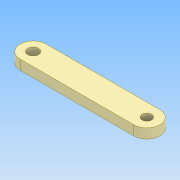
# Autodesk Inventor part: Selection_Counterweight
Saved by Autodesk Inventor 2018.1 (Build 221171000, 171)
## iProperties
Created: 2019-02-14
Part Number: Selection_Counterweight
Material: Nylon 6/6
Document SubType Name: Modeling
Designer: James
Density: 1.13 g/cm^3
Appearance: Nylon 6
Author: James
Autodesk Inventor part; units mm, degrees
ref_plane "YZ Plane" through (0, 0, 0) normal (1, 0, 0) x (0, 1, 0)
ref_plane "XZ Plane" through (0, 0, 0) normal (0, 1, 0) x (-1, 0, 0)
ref_plane "XY Plane" through (0, 0, 0) normal (0, 0, 1) x (1, 0, 0)
sketch "Sketch1" plane through (0, 0, 0) normal (0, 0, 1) x (1, 0, 0)
  circle A0 centre (0, 0) radius 4
  circle A1 centre (-35, 0) radius 4
  line L0 (-35, 4) -> (0, 4)
  line L1 (0, -4) -> (-35, -4)
  dimension "d0" = 8
  dimension "d1" = 8
  dimension "d2" = 35
  constraints: 4 end point, 4 point on circle, 4 tangent, 2 centre point, 1 coincident, 1 horizontal alignment
  measures "d0" diameter of A0
  measures "d1" diameter of A1
  measures "d2" distance of point (0, 0) A1.centre
extrude "Extrusion1" add sketch "Sketch1" along normal blind 3
sketch "Sketch3" plane through (0, 0, 3) normal (0, 0, 1) x (1, 0, 0)
  arc A0 (-35, 4) -> (-35, -4) centre (-35, 0) ccw projected
  line L0 (-35, -4) -> (0, -4) projected
  arc A1 (0, -4) -> (0, 4) centre (0, 0) ccw projected
  line L1 (0, 4) -> (-35, 4) projected
  constraints: 1 coincident
hole "Hole1" at (0, 0, 3) direction (0, 0, -1) diameter 3 end through all
sketch "Sketch4" plane through (0, 0, 3) normal (0, 0, 1) x (1, 0, 0)
  circle A0 centre (0, 0) radius 1.5 projected
  arc A1 (-35, 4) -> (-35, -4) centre (-35, 0) ccw projected
  line L0 (-35, -4) -> (0, -4) projected
  arc A2 (0, -4) -> (0, 4) centre (0, 0) ccw projected
  line L1 (0, 4) -> (-35, 4) projected
  constraints: 1 coincident
hole "Hole2" at (-35, 0, 3) direction (0, 0, -1) diameter 3.4 end through all clearance for "Socket Head Cap Screw" size "M3" standard "Ansi Metric M Profile"
body "Solid1"
